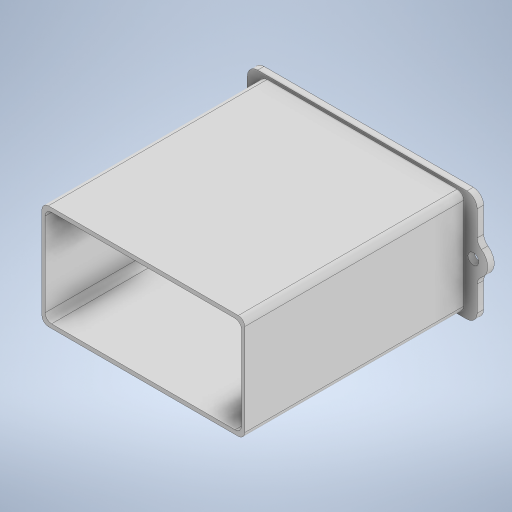
# Autodesk Inventor part: нижняя часть держателя аккумов
Saved by Autodesk Inventor 2023.1 (Build 271208000, 208)
## iProperties
Created: 2023-02-22
Part Number: нижняя часть держателя аккумов
Material: Типовые
Document SubType Name: Modeling
Designer: User
Density: 1 g/cm^3
Appearance: По умолчанию
Author: User
Autodesk Inventor part; units mm, degrees
ref_plane "YZ Plane" through (0, 0, 0) normal (1, 0, 0) x (0, 1, 0)
ref_plane "XZ Plane" through (0, 0, 0) normal (0, 1, 0) x (-1, 0, 0)
ref_plane "XY Plane" through (0, 0, 0) normal (0, 0, 1) x (1, 0, 0)
sketch "Эскиз1" plane through (0, 0, 0) normal (0, 0, 1) x (1, 0, 0)
  line L0 (-30.5, 15) -> (30.5, 15)
  line L1 (30.5, 15) -> (30.5, -15)
  line L2 (30.5, -15) -> (-30.5, -15)
  line L3 (-30.5, -15) -> (-30.5, 15)
  line L4 (0, -24.15) -> (0, 24.15) projected
  line L5 (-45.5, 0) -> (45.5, 0) projected
  line L6 (-32.5, 17.25) -> (32.5, 17.25)
  line L7 (32.5, 17.25) -> (32.5, -17.25)
  line L8 (32.5, -17.25) -> (-32.5, -17.25)
  line L9 (-32.5, -17.25) -> (-32.5, 17.25)
  point P0 (0, 0)
  dimension "d0" = 61
  dimension "d1" = 30
  dimension "d2" = 34.5
  dimension "d3" = 65
  constraints: 16 end point, 4 parallel, 2 horizontal, 2 perpendicular, 4 other
  measures "d0" distance between parallel lines of L1 L3
  measures "d1" distance between parallel lines of L2 L0
  measures "d2" distance between parallel lines of L8 L6
  measures "d3" distance between parallel lines of L7 L9
extrude "Выдавливание1" add sketch "Эскиз1" along normal blind 3
extrude "Выдавливание2" add sketch "Эскиз1" against normal blind 80 contours L3 L5 L9 L6 L4 L0 | L4 L6 L7 L5 L1 L0 | L3 L2 L4 L8 L9 L5 | L5 L7 L8 L4 L2 L1
sketch "Эскиз2" plane through (0, 0, 3) normal (0, 0, 1) x (1, 0, 0)
  circle A0 centre (-10, 0) radius 5.6
  circle A1 centre (10, 0) radius 5.6
  line L0 (0, -24.15) -> (0, 24.15) projected
  point P0 (0, 0)
  dimension "d8" = 20
  dimension "d9" = 11.2
  dimension "d10" = 11.2
  constraints: 2 centre point, 1 symmetric about line
  measures "d8" distance of A1.centre A0.centre
  measures "d9" diameter of A0
  measures "d10" diameter of A1
extrude "Выдавливание3" cut sketch "Эскиз2" against normal blind 80
sketch "Эскиз3" plane through (0, 0, -80) normal (0, 0, -1) x (-1, 0, 0)
  line L0 (30.5, -15) -> (-30.5, -15) projected
  circle A0 centre (-10, 0) radius 5.6 projected
  circle A1 centre (10, 0) radius 5.6 projected
  line L1 (-30.5, -15) -> (30.5, -15) projected
  line L2 (30.5, -15) -> (30.5, 15) projected
  line L3 (30.5, 15) -> (-30.5, 15) projected
  line L4 (-30.5, 15) -> (-30.5, -15) projected
  line L5 (32.5, -17.25) -> (-32.5, -17.25)
  line L6 (-35.7, -14.05) -> (-35.7, 14.05)
  line L7 (-32.5, 17.25) -> (32.5, 17.25)
  line L8 (35.7, 14.05) -> (35.7, -14.05)
  line L9 (0, -28.8249) -> (0, 30.0984) projected
  line L10 (57.8663, 0) -> (-57.8663, 0) projected
  line L11 (32.5, -17.25) -> (32.5, 17.25) projected
  line L12 (-32.5, 17.25) -> (-32.5, -17.25) projected
  arc A2 (32.5, -17.25) -> (35.7, -14.05) centre (32.5, -14.05) ccw
  arc A3 (35.7, 14.05) -> (32.5, 17.25) centre (32.5, 14.05) ccw
  arc A4 (-32.5, 17.25) -> (-35.7, 14.05) centre (-32.5, 14.05) ccw
  arc A5 (-35.7, -14.05) -> (-32.5, -17.25) centre (-32.5, -14.05) ccw
  point P0 (0, 0)
  point P1 (35.7, -17.25)
  point P2 (-30.5, -15)
  dimension "d13" = 3.2
  dimension "d14" = 3.2
  dimension "d15" = 3.2
  constraints: 8 end point, 8 point on circle, 8 tangent, 4 centre point, 3 equal radius, 2 parallel, 2 point on line, 1 horizontal, 1 horizontal alignment, 1 perpendicular, 2 other
  measures "d13" distance between parallel lines of L8 L11
  measures "d14" distance between parallel lines of L6 L12
  measures "d15" radius of A2
extrude "Выдавливание4" add sketch "Эскиз3" along normal blind 2 contours L2 L10 L11 L5 L9 L0 | L9 L5 L12 L10 L4 L0 | L2 L3 L9 L7 L11 L10 | L11 A3 L8 L10 | L10 L8 A2 L11 | L10 L12 L7 L9 L3 L4 | A5 L6 L10 L12 | L10 L6 A4 L12
sketch "Эскиз4" plane through (0, 0, -82) normal (0, 0, -1) x (-1, 0, 0)
  line L0 (35.7, -14.05) -> (35.7, 14.05) projected
  arc A0 (35.7, -3.2879) -> (35.7, 3.2879) centre (34.5, 0) ccw
  line L1 (30.5, 15) -> (30.5, -15) projected
  arc A1 (35.7, -4.337) -> (35.7, 4.337) centre (34.5, 0) ccw
  line L2 (0, 0) -> (0, 3.9976)
  line L3 (-35.7, 14.05) -> (-35.7, -14.05) projected
  arc A2 (-35.7, 3.2879) -> (-35.7, -3.2879) centre (-34.5, 0) ccw
  arc A3 (-35.7, 4.337) -> (-35.7, -4.337) centre (-34.5, 0) ccw
  circle A4 centre (34.5, 0) radius 1.7
  circle A5 centre (-34.5, 0) radius 1.7
  point P0 (28.7, 0)
  point P1 (30.5, 0)
  point P2 (31, 0)
  point P3 (-35.7, -4.4956)
  point P4 (-35.7, 4.4956)
  dimension "d19" = 7
  dimension "d20" = 4
  dimension "d21" = 1
  dimension "d26" = 3.4
  dimension "d27" = 3.4
  constraints: 9 point on circle, 6 centre point, 6 point on line, 6 symmetric about line, 4 coincident, 2 end point, 1 midpoint, 1 vertical, 2 other
  measures "d19" diameter of A0
  measures "d20" distance of point (30.5, 0) A0.centre
  measures "d21" radial gap between concentric circles of A1 A0
  measures "d26" diameter of A4
  measures "d27" diameter of A5
extrude "Выдавливание5" add sketch "Эскиз4" against normal blind 2 contours L0 A0 A1 | L0 A4 A0 | L0 A4 picked at (35.8557, 0.1108)
extrude "Выдавливание6" add sketch "Эскиз4" against normal blind 2 contours L3 A2 A3 | L3 A5 A2 | L3 A5 picked at (-35.7794, -0.3021)
extrude "Выдавливание7" cut sketch "Эскиз4" against normal blind 2 contours A4 L0 | L0 A4 | A5 L3 | L3 A5
fillet "Сопряжение1" radius 3 4 edges at (35.7, -4.337, -81) (35.7, 4.337, -81) (-35.7, -4.337, -81) (-35.7, 4.337, -81)
sketch "Эскиз5" plane through (0, 0, 3) normal (0, 0, 1) x (1, 0, 0)
  line L0 (32.5, 17.25) -> (-32.5, 17.25) projected
  circle A0 centre (10, 0) radius 5.6 projected
  circle A1 centre (-10, 0) radius 5.6 projected
  line L1 (32.5, 17.25) -> (-32.5, 17.25) projected
  line L2 (-32.5, 17.25) -> (-32.5, -17.25) projected
  line L3 (-32.5, -17.25) -> (32.5, -17.25) projected
  line L4 (32.5, -17.25) -> (32.5, 17.25) projected
  point P0 (0, 0)
extrude "Выдавливание8" cut sketch "Эскиз5" against normal up to surface (3 mm away) contours L4 L3 L2 L0 | A0 | A1
sketch "Эскиз6" plane through (-32.5, -17.25, 0) normal (0, 0, 1) x (1, 0, 0)
  line L0 (63, 2.25) -> (2, 2.25) projected
  line L1 (2, 2.25) -> (2, 32.25) projected
  line L2 (2, 32.25) -> (63, 32.25) projected
  line L3 (63, 32.25) -> (63, 2.25) projected
  line L4 (0, 0) -> (0, 34.5) projected
  line L5 (65, 0) -> (0, 0) projected
  line L6 (65, 34.5) -> (65, 0) projected
  line L7 (0, 34.5) -> (65, 34.5) projected
  point P0 (32.5, 17.25)
extrude "Выдавливание9" cut sketch "Эскиз1" against normal blind 12 contours L3 L5 L9 L6 L4 L0 | L4 L6 L7 L5 L1 L0 | L3 L2 L4 L8 L9 L5 | L5 L7 L8 L4 L2 L1
sketch "Эскиз7" plane through (0, 0, -12) normal (0, 0, 1) x (1, 0, 0)
  line L0 (-32.5, 17.25) -> (32.5, 17.25) projected
  line L1 (-32.5, 17.25) -> (32.5, 17.25) projected
  line L2 (-32.5, -17.25) -> (-32.5, 17.25) projected
  line L3 (32.5, -17.25) -> (-32.5, -17.25) projected
  line L4 (32.5, 17.25) -> (32.5, -17.25) projected
  line L5 (30.5, -15) -> (30.5, 15) projected
  line L6 (-30.5, -15) -> (30.5, -15) projected
  line L7 (-30.5, 15) -> (-30.5, -15) projected
  line L8 (30.5, 15) -> (-30.5, 15) projected
  line L9 (-31.5, 16.25) -> (31.5, 16.25)
  line L10 (31.5, 16.25) -> (31.5, -16.25)
  line L11 (31.5, -16.25) -> (-31.5, -16.25)
  line L12 (-31.5, -16.25) -> (-31.5, 16.25)
  point P0 (0, 0)
  dimension "d35" = 1
  dimension "d36" = 1
  dimension "d37" = 1
  dimension "d38" = 1
  constraints: 8 end point, 2 parallel, 1 horizontal, 1 perpendicular
  measures "d35" distance between parallel lines of L9 L0
  measures "d36" distance between parallel lines of L2 L12
  measures "d37" distance between parallel lines of L3 L11
  measures "d38" distance between parallel lines of L4 L10
extrude "Выдавливание10" cut sketch "Эскиз7" against normal up to surface (68 mm away) contours L0 L4 L3 L2
fillet "Сопряжение2" radius 2 8 edges at (31.5, 16.25, -46) (30.5, 15, -47) (30.5, -15, -47) (31.5, -16.25, -46) (-31.5, -16.25, -46) (-31.5, 16.25, -46) (-30.5, -15, -47) (-30.5, 15, -47)
